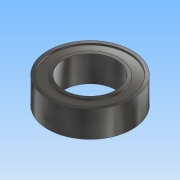
# Autodesk Inventor part: MR85 ZZ
Saved by Autodesk Inventor 2017 (Build 210142000, 142)
## iProperties
Part Number: MR85 ZZ
Material: Типовые
Document SubType Name: Modeling
Designer: STALKER
Density: 1 g/cm^3
Appearance: Сталь - гальванизированная
Author: STALKER
Autodesk Inventor part; units mm, degrees
ref_plane "YZ Plane" through (0, 0, 0) normal (1, 0, 0) x (0, 1, 0)
ref_plane "XZ Plane" through (0, 0, 0) normal (0, 1, 0) x (-1, 0, 0)
ref_plane "XY Plane" through (0, 0, 0) normal (0, 0, 1) x (1, 0, 0)
sketch "Эскиз1" plane through (0, 0, 0) normal (0, 0, 1) x (1, 0, 0)
  circle A0 centre (0, 0) radius 4
  circle A1 centre (0, 0) radius 2.5
  circle A2 centre (0, 0) radius 3.7
  circle A3 centre (0, 0) radius 2.8
  dimension "d0" = 8
  dimension "d1" = 5
  dimension "d2" = 0.3
  dimension "d3" = 0.3
  constraints: 4 centre point, 4 coincident
  measures "d0" diameter of A0
  measures "d1" diameter of A1
  measures "d2" radial gap between concentric circles of A2 A0
  measures "d3" radial gap between concentric circles of A1 A3
extrude "Выдавливание1" add sketch "Эскиз1" along normal mid plane 2.5
extrude "Выдавливание2" add sketch "Эскиз1" along normal mid plane 2.2 contours A2
